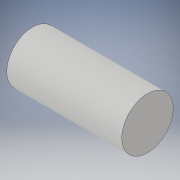
# Autodesk Inventor part: PLTW 6.5
Saved by Autodesk Inventor 2017 (Build 210142000, 142)
## iProperties
Created: 2017-03-01
Part Number: PLTW 6.5
Material: Generic
Document SubType Name: Modeling
Designer: rbibb
Density: 1 g/cm^3
Appearance: Default
Author: rbibb
Autodesk Inventor part; units mm, degrees
ref_plane "YZ Plane" through (0, 0, 0) normal (1, 0, 0) x (0, 1, 0)
ref_plane "XZ Plane" through (0, 0, 0) normal (0, 1, 0) x (-1, 0, 0)
ref_plane "XY Plane" through (0, 0, 0) normal (0, 0, 1) x (1, 0, 0)
sketch "Sketch1" plane through (0, 0, 0) normal (1, 0, 0) x (0, 1, 0)
  circle A0 centre (9.4093, 19.9136) radius 5.6793
  point P0 (0, 0)
  dimension "d0" = 25.4
  constraints: 1 centre point
extrude "Extrusion1" add sketch "Sketch1" along normal blind 25.4
body "Solid1"
